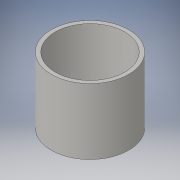
# Autodesk Inventor part: button_bottom
Saved by Autodesk Inventor 2016 SP2 (Build 200236200, 236)
## iProperties
Created: 2017-09-04
Part Number: button_bottom
Material: Generic
Document SubType Name: Modeling
Designer: Kartikye
Density: 1 g/cm^3
Appearance: Default
Author: Kartikye
Autodesk Inventor part; units mm, degrees
ref_plane "YZ Plane" through (0, 0, 0) normal (1, 0, 0) x (0, 1, 0)
ref_plane "XZ Plane" through (0, 0, 0) normal (0, 1, 0) x (-1, 0, 0)
ref_plane "XY Plane" through (0, 0, 0) normal (0, 0, 1) x (1, 0, 0)
sketch "Sketch1" plane through (0, 0, 0) normal (0, 1, 0) x (-1, 0, 0)
  circle A0 centre (0, 0) radius 5
  dimension "d0" = 10
  constraints: 1 centre point, 1 coincident
  measures "d0" diameter of A0
sketch "Sketch2" plane through (0, 0, 0) normal (0, 1, 0) x (-1, 0, 0)
  point P0 (0, 0)
extrude "Extrusion1" add sketch "Sketch1" along normal blind 1.5
sketch "Sketch3" plane through (0, 1.5, 0) normal (0, 1, 0) x (1, 0, 0)
  circle A0 centre (0, 0) radius 4.5
  circle A1 centre (0, 0) radius 5
  dimension "d3" = 9
  constraints: 2 centre point, 1 coincident
  measures "d3" diameter of A0
extrude "Extrusion2" add sketch "Sketch3" along normal blind 7
sketch "Sketch4" plane through (0, 1.5, 0) normal (0, 1, 0) x (1, 0, 0)
  line L0 (3, 3) -> (3.5, 3)
  line L1 (3.5, 3) -> (3.5, 2)
  line L2 (3.5, 2) -> (3, 2)
  line L3 (3, 2) -> (3, 3)
  line L4 (3, 3) -> (3.5, 2) construction
  line L5 (3.5, 3) -> (3, 2) construction
  line L6 (-3.5, 3) -> (-3, 3)
  line L7 (-3, 3) -> (-3, 2)
  line L8 (-3, 2) -> (-3.5, 2)
  line L9 (-3.5, 2) -> (-3.5, 3)
  line L10 (-3.5, 3) -> (-3, 2) construction
  line L11 (-3, 3) -> (-3.5, 2) construction
  line L12 (-3.5, -2) -> (-3, -2)
  line L13 (-3, -2) -> (-3, -3)
  line L14 (-3, -3) -> (-3.5, -3)
  line L15 (-3.5, -3) -> (-3.5, -2)
  line L16 (-3.5, -2) -> (-3, -3) construction
  line L17 (-3, -2) -> (-3.5, -3) construction
  line L18 (3, -2) -> (3.5, -2)
  line L19 (3.5, -2) -> (3.5, -3)
  line L20 (3.5, -3) -> (3, -3)
  line L21 (3, -3) -> (3, -2)
  point P0 (0, 0)
  point P1 (3.25, 2.5)
  point P2 (-3.25, 2.5)
  point P3 (-3.25, -2.5)
  dimension "d8" = 0.5
  dimension "d9" = 1
  dimension "d10" = 0.5
  dimension "d11" = 1
  dimension "d12" = 0.5
  dimension "d13" = 1
  dimension "d15" = 6
  dimension "d16" = 7
  dimension "d17" = 0
  dimension "d18" = 0
  dimension "d20" = 0.5
  dimension "d21" = 1
  dimension "d22" = 7
  dimension "d23" = 0
  dimension "d24" = 3.5
  dimension "d26" = 3
  constraints: 44 end point, 8 parallel, 6 midpoint, 4 horizontal, 4 perpendicular
  measures "d8" distance of L1.end L2.end
  measures "d9" distance of L0.end L1.end
  measures "d10" distance of L7.end L8.end
  measures "d11" distance of L6.end L7.end
  measures "d12" distance of L13.end L14.end
  measures "d13" distance of L12.end L13.end
  measures "d15" distance between parallel lines of L14 L6
  measures "d16" distance between parallel lines of L9 L1
  measures "d17" distance between parallel lines of L9 L15
  measures "d18" distance between parallel lines of L6 L0
  measures "d20" distance of L19.end L20.end
  measures "d21" distance of L18.end L19.end
  measures "d22" distance between parallel lines of L15 L19
  measures "d23" distance between parallel lines of L14 L20
  measures "d24" distance from line of point (0, 0) L15
  measures "d26" distance from line of point (0, 0) L20
extrude "Extrusion3" cut sketch "Sketch4" against normal blind 7
body "Solid1"
